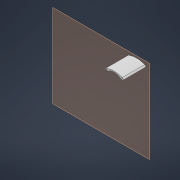
# Autodesk Inventor part: foot_01
Saved by Autodesk Inventor 2022 (Build 260153000, 153)
## iProperties
Created: 2025-02-06
Part Number: foot_01
Material: 一般
Document SubType Name: Modeling
Designer: gisen
Density: 1 g/cm^3
Appearance: 既定
Author: gisen
Autodesk Inventor part; units mm, degrees
ref_plane "YZ Plane" through (0, 0, 0) normal (1, 0, 0) x (0, 1, 0)
ref_plane "XZ Plane" through (0, 0, 0) normal (0, 1, 0) x (-1, 0, 0)
ref_plane "XY Plane" through (0, 0, 0) normal (0, 0, 1) x (1, 0, 0)
ref_plane "作業平面1" through (0, 0, 0) normal (0, 0, 1) x (1, 0, 0)
sketch "スケッチ1" plane through (0, 0, 0) normal (0, 0, 1) x (1, 0, 0)
  circle A0 centre (250, 230) radius 3 construction
  line L0 (246.124, 222.5) -> (255, 222.5) construction
  circle A1 centre (239, 219) radius 3 construction
  circle A2 centre (161.1336, 230) radius 3 construction
  arc A3 (-159.3342, 234.665) -> (159.3342, 234.665) centre (0, 647.734) ccw construction
  line L1 (250, 235) -> (161.1336, 235) construction
  circle A4 centre (250, 230) radius 3.2
  circle A5 centre (161.1336, 230) radius 3.2
  circle A6 centre (250, 230) radius 7.5 construction
  circle A7 centre (161.1336, 230) radius 7.5 construction
  line L2 (250, 230) -> (161.1336, 230) construction
  line L3 (205.5668, 230) -> (205.5668, 246) construction
  arc A8 (252.7682, 236.9705) -> (158.3654, 236.9705) centre (205.5668, 118.1142) ccw
  arc A9 (243.602, 233.9135) -> (167.5316, 233.9135) centre (205.5668, 118.1142) ccw
  arc A10 (243.602, 233.9135) -> (252.7682, 236.9705) centre (250, 230) ccw
  arc A11 (158.3654, 236.9705) -> (167.5316, 233.9135) centre (161.1336, 230) ccw
  point P0 (0, 0)
  dimension "d0" = 6.4
  dimension "d1" = 15
  dimension "d2" = 16
  dimension "d3" = 6
  constraints: 13 point on circle, 8 centre point, 6 coincident, 4 end point, 2 equal radius, 2 tangent, 1 horizontal, 1 midpoint, 1 vertical
  measures "d0" diameter of A4
  measures "d1" diameter of A6
  measures "d2" distance of L3.start L3.end
  measures "d3" radial gap between concentric circles of A8 A9
extrude "押し出し1" add sketch "スケッチ1" along normal blind 130
fillet "フィレット1" radius 60 2 edges at (243.602, 233.9135, 65) (167.5316, 233.9135, 65)
sketch "スケッチ2" plane through (0, 0, 0) normal (0, 0, -1) x (-1, 0, 0)
  arc A0 (-166.1782, 224.45) -> (-158.3654, 236.9705) centre (-161.1336, 230) ccw projected
  circle A1 centre (-161.1336, 230) radius 3.2 projected
  circle A2 centre (-250, 230) radius 3.2 projected
  circle A3 centre (-250, 230) radius 88.8664 construction
  arc A4 (-158.4511, 222.9961) -> (-158.1923, 228.7397) centre (-250, 230) ccw
  arc A5 (-164.3511, 223.2252) -> (-164.0923, 228.7808) centre (-250, 230) ccw
  point P0 (0, 0)
  dimension "d7" = 2.95
  dimension "d8" = 2.95
  constraints: 8 point on circle, 3 coincident, 2 centre point, 1 horizontal alignment, 2 other
extrude "押し出し2" cut sketch "スケッチ2" against normal through all contours A5 A1 A4 A0
fillet "フィレット2" radius 2 4 edges at (158.4511, 222.9961, 65) (164.3511, 223.2252, 65) (164.0923, 228.7808, 65) (158.1923, 228.7397, 65)
equation "\"d8\" = d7"
